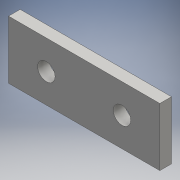
# Autodesk Inventor part: prepoj
Saved by Autodesk Inventor 2016 (Build 200138000, 138)
## iProperties
Created: 2016-01-30
Part Number: prepoj
Material: Generic
Document SubType Name: Modeling
Designer: Juraj
Density: 1 g/cm^3
Appearance: Default
Author: Juraj
Autodesk Inventor part; units mm, degrees
ref_plane "YZ Plane" through (0, 0, 0) normal (1, 0, 0) x (0, 1, 0)
ref_plane "XZ Plane" through (0, 0, 0) normal (0, 1, 0) x (-1, 0, 0)
ref_plane "XY Plane" through (0, 0, 0) normal (0, 0, 1) x (1, 0, 0)
sketch "Sketch1" plane through (0, 0, 0) normal (0, 1, 0) x (-1, 0, 0)
  line L0 (3.1278, 4.0625) -> (3.1278, -5.9375)
  line L1 (3.1278, -5.9375) -> (-22.8722, -5.9375)
  line L2 (-22.8722, -5.9375) -> (-22.8722, 4.0625)
  line L3 (-22.8722, 4.0625) -> (3.1278, 4.0625)
  circle A0 centre (-3.3722, -0.9375) radius 1.5
  line L4 (-9.8722, -5.9375) -> (-9.8722, 8.6537)
  circle A1 centre (-16.3722, -0.9375) radius 1.5
  point P0 (0, 0)
  dimension "d0" = 10
  dimension "d1" = 26
  dimension "d2" = 3
  dimension "d4" = 6.5
  dimension "d5" = 6.5
  dimension "d6" = 13
  constraints: 10 end point, 3 perpendicular, 2 centre point, 2 vertical, 1 midpoint, 1 symmetric about line, 1 other
  measures "d0" distance of L0.start L0.end
  measures "d1" distance of L0.end L1.end
  measures "d2" diameter of A0
  measures "d4" distance from line of L0 A0.centre
  measures "d5" distance from line of L4 A0.centre
  measures "d6" distance between parallel lines of L0 L4
extrude "Extrusion1" add sketch "Sketch1" along normal blind 2
body "Solid1"
